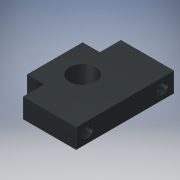
# Autodesk Inventor part: Loslager
Saved by Autodesk Inventor 2019 (Build 230136000, 136)
## iProperties
Created: 2021-04-25
Part Number: Loslager
Material: Eisen, Grau
Document SubType Name: Modeling
Designer: Michael Sumper
Density: 7.15 g/cm^3
Appearance: Eisen - Grau
Author: Michael Sumper
Autodesk Inventor part; units mm, degrees
ref_plane "YZ Plane" through (0, 0, 0) normal (1, 0, 0) x (0, 1, 0)
ref_plane "XZ Plane" through (0, 0, 0) normal (0, 1, 0) x (-1, 0, 0)
ref_plane "XY Plane" through (0, 0, 0) normal (0, 0, 1) x (1, 0, 0)
sketch "Skizze1" plane through (0, 0, 0) normal (0, 1, 0) x (-1, 0, 0)
  line L0 (0, 0) -> (0, -60)
  line L1 (0, -60) -> (32.5, -60)
  line L2 (32.5, -60) -> (32.5, -47)
  line L3 (32.5, -47) -> (43, -47)
  line L4 (43, -47) -> (43, -13)
  line L5 (43, -13) -> (32.5, -13)
  line L6 (32.5, -13) -> (32.5, 0)
  line L7 (32.5, 0) -> (0, 0)
  dimension "d0" = 60
  dimension "d1" = 32.5
  dimension "d2" = 13
  dimension "d3" = 10.5
  dimension "d4" = 34
  dimension "d5" = 10.5
  dimension "d6" = 13
  constraints: 16 end point, 4 perpendicular, 2 point on line, 1 vertical
  measures "d0" distance of L0.start L0.end
  measures "d1" distance of L0.end L1.end
  measures "d2" distance of L1.end L2.end
  measures "d3" distance of L2.end L3.end
  measures "d4" distance of L3.end L4.end
  measures "d5" distance of L4.end L5.end
  measures "d6" distance of L5.end L6.end
extrude "Extrusion1" add sketch "Skizze1" along normal blind 12
sketch "Skizze2" plane through (-32.5, 0, -60) normal (-1, 0, 0) x (0, 0, 1)
  line L0 (0, 0) -> (13, 0) construction
  line L1 (13, 0) -> (13, 12) construction
  line L2 (0, 12) -> (13, 12) construction
  line L3 (0, 0) -> (0, 12) construction
  line L4 (47, 0) -> (60, 0) construction
  line L5 (60, 0) -> (60, 12) construction
  line L6 (47, 12) -> (60, 12) construction
  line L7 (47, 0) -> (47, 12) construction
  line L8 (60, 12) -> (0, 12) construction
  line L9 (0, 12) -> (0, 6) construction
  line L10 (0, 0) -> (0, 12) construction
  line L11 (0, 6) -> (7, 6) construction
  line L12 (7, 6) -> (53, 6) construction
  dimension "d9" = 6
  dimension "d10" = 7
  dimension "d11" = 46
  constraints: 6 end point, 1 midpoint, 1 perpendicular, 1 point on line
  measures "d9" distance of L2.start L9.end
  measures "d10" distance of L9.end L11.end
  measures "d11" distance of L11.end L12.end
hole "Bohrung1" at (-32.5, 6, -53) at (-32.5, 6, -7) direction (1, 0, 0) diameter 6.6 end through all counterbore diameter 11 counterbore depth 6 clearance for "Innensechskantkopfschraube" size "M6" standard "ANSI Metrisches M Profil"
sketch "Skizze3" plane through (0, 12, 0) normal (0, 1, 0) x (1, 0, 0)
  line L0 (-32.5, 47) -> (-43, 47) construction
  line L1 (-43, 47) -> (-9, 47) construction
  line L2 (-9, 47) -> (-9, 13) construction
  line L3 (-9, 13) -> (-43, 13) construction
  line L4 (-43, 13) -> (-43, 47) construction
  line L5 (-9, 30) -> (-43, 30) construction
  line L6 (-43, 47) -> (-43, 13) construction
  line L7 (-26, 47) -> (-26, 13) construction
  point P0 (0, 0)
  dimension "d19" = 34
  dimension "d20" = 34
  constraints: 12 end point, 4 midpoint, 2 parallel, 1 horizontal, 1 perpendicular
  measures "d19" distance of L2.end L3.end
  measures "d20" distance of L1.end L2.end
sketch "Skizze4" plane through (0, 12, 0) normal (0, 1, 0) x (1, 0, 0)
  point P0 (0, 0)
  point P1 (-26, 30)
hole "Bohrung2" at (-26, 12, -30) direction (0, -1, 0) diameter 16 end through all
